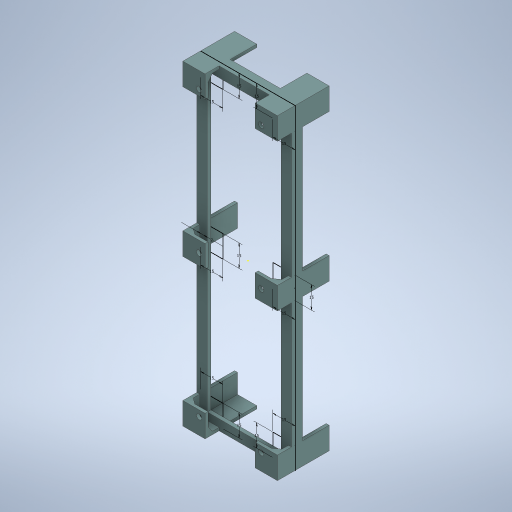
# Autodesk Inventor part: BaseMotor
Saved by Autodesk Inventor 2024 (Build 280153000, 153)
## iProperties
Created: 2024-02-15
Part Number: BaseMotor
Material: Generic
Document SubType Name: Modeling
Designer: fabiancastano
Density: 1 g/cm^3
Appearance: Default
Author: fabiancastano
Autodesk Inventor part; units mm, degrees
ref_plane "YZ Plane" through (0, 0, 0) normal (1, 0, 0) x (0, 1, 0)
ref_plane "XZ Plane" through (0, 0, 0) normal (0, 1, 0) x (-1, 0, 0)
ref_plane "XY Plane" through (0, 0, 0) normal (0, 0, 1) x (1, 0, 0)
sketch "Sketch1" plane through (0, 0, 0) normal (0, 0, 1) x (1, 0, 0)
  line L0 (-30, -105) -> (-30, 105) projected
  line L1 (-30, 105) -> (30, 105) projected
  line L2 (30, 105) -> (30, -105) projected
  line L3 (30, -105) -> (-30, -105) projected
  line L4 (-32, 107) -> (-32, -107)
  line L5 (-32, -107) -> (32, -107)
  line L6 (32, -107) -> (32, 107)
  line L7 (32, 107) -> (-32, 107)
  line L8 (-30, 105) -> (30, 105)
  line L9 (30, 105) -> (30, -105)
  line L10 (30, -105) -> (-30, -105)
  line L11 (-30, -105) -> (-30, 105)
  line L12 (-32, 107) -> (-17, 107)
  line L13 (-17, 107) -> (-17, 92)
  line L14 (-17, 92) -> (-32, 92)
  line L15 (-32, 92) -> (-32, 107)
  line L16 (32, 107) -> (17, 107)
  line L17 (17, 107) -> (17, 92)
  line L18 (17, 92) -> (32, 92)
  line L19 (32, 92) -> (32, 107)
  line L20 (32, -107) -> (17, -107)
  line L21 (17, -107) -> (17, -92)
  line L22 (17, -92) -> (32, -92)
  line L23 (32, -92) -> (32, -107)
  line L24 (-32, -107) -> (-17, -107)
  line L25 (-17, -107) -> (-17, -92)
  line L26 (-17, -92) -> (-32, -92)
  line L27 (-32, -92) -> (-32, -107)
  line L28 (17, 7.5) -> (32, 7.5)
  line L29 (32, 7.5) -> (32, -7.5)
  line L30 (32, -7.5) -> (17, -7.5)
  line L31 (17, -7.5) -> (17, 7.5)
  line L32 (-32, 7.5) -> (-17, 7.5)
  line L33 (-17, 7.5) -> (-17, -7.5)
  line L34 (-17, -7.5) -> (-32, -7.5)
  line L35 (-32, -7.5) -> (-32, 7.5)
  point P0 (0, 0)
  point P1 (-32, 0)
  point P2 (-32, 0)
  point P3 (32, 0)
  point P4 (32, 0)
  point P5 (-30, -7.5)
  point P6 (-30, 7.5)
  point P7 (30, -7.5)
  point P8 (30, 7.5)
  point P9 (-30, -92)
  point P10 (-17, -105)
  point P11 (30, -92)
  point P12 (17, -105)
  point P13 (30, 92)
  point P14 (17, 105)
  point P15 (-30, 92)
  point P16 (-17, 105)
  dimension "d0" = 2
  dimension "d1" = 15
  dimension "d2" = 15
  dimension "d3" = 15
  dimension "d4" = 15
  dimension "d5" = 15
  dimension "d6" = 15
  dimension "d7" = 15
  dimension "d8" = 15
  dimension "d9" = 15
  dimension "d10" = 15
  dimension "d11" = 15
  dimension "d12" = 15
  constraints: 64 end point, 14 parallel, 7 horizontal, 7 perpendicular, 4 coincident, 4 midpoint, 3 other
  measures "d0" distance between parallel lines of L0 L4
  measures "d1" distance of L13.end L14.end
  measures "d2" distance of L12.end L13.end
  measures "d3" distance of L18.end L17.end
  measures "d4" distance of L17.end L16.end
  measures "d5" distance of L21.end L22.end
  measures "d6" distance of L20.end L21.end
  measures "d7" distance of L26.end L25.end
  measures "d8" distance of L25.end L24.end
  measures "d9" distance of L29.end L30.end
  measures "d10" distance of L28.end L29.end
  measures "d11" distance of L33.end L34.end
  measures "d12" distance of L32.end L33.end
extrude "Extrusion1" add sketch "Sketch1" against normal blind 23 contours L3 L25 L5 L4 L26 L0 | L34 L4 L32 L0 | L3 L2 L22 L6 L5 L21 | L14 L4 L7 L13 L1 L0 | L2 L28 L6 L30 | L17 L7 L6 L18 L2 L1
sketch "Sketch2" plane through (0, 0, 0) normal (0, 0, 1) x (1, 0, 0)
  line L0 (17, 107) -> (17, 105) projected
  line L1 (17, 105) -> (17, 107) projected
  line L2 (17, 107) -> (17, 105) projected
  line L3 (17, 105) -> (17, 107) projected
  line L4 (30, 105) -> (17, 105) projected
  line L5 (17, 105) -> (30, 105) projected
  line L6 (30, 105) -> (17, 105) projected
  line L7 (30, 92) -> (30, 105) projected
  line L8 (30, 105) -> (30, 92) projected
  line L9 (30, 92) -> (30, 105) projected
  line L10 (17, 107) -> (32, 107) projected
  line L11 (32, 107) -> (17, 107) projected
  line L12 (17, 107) -> (32, 107) projected
  line L13 (32, 107) -> (32, 92) projected
  line L14 (32, 92) -> (32, 107) projected
  line L15 (32, 107) -> (32, 92) projected
  line L16 (32, 107) -> (32, 92) projected
  line L17 (32, 92) -> (30, 92) projected
  line L18 (30, 92) -> (30, 105) projected
  line L19 (30, 105) -> (17, 105) projected
  line L20 (17, 105) -> (17, 107) projected
  line L21 (17, 107) -> (32, 107) projected
  line L22 (17, 105) -> (30, 105) projected
  line L23 (32, 107) -> (17, 107) projected
  line L24 (32, 92) -> (32, 107) projected
  line L25 (32, 107) -> (17, 107) projected
  line L26 (17, 107) -> (17, 105) projected
  line L27 (17, 105) -> (30, 105) projected
  line L28 (30, 105) -> (30, 92) projected
  line L29 (30, 92) -> (32, 92) projected
  line L30 (32, 92) -> (32, 107) projected
  line L31 (-30, -7.5) -> (-30, 7.5) projected
  line L32 (-30, -7.5) -> (-30, 7.5) projected
  line L33 (-30, 7.5) -> (-30, -7.5) projected
  line L34 (-32, -7.5) -> (-30, -7.5) projected
  line L35 (-30, 7.5) -> (-32, 7.5) projected
  line L36 (-32, 7.5) -> (-32, -7.5) projected
  line L37 (-32, 7.5) -> (-32, -7.5) projected
  line L38 (-32, -7.5) -> (-32, 7.5) projected
  line L39 (-32, -7.5) -> (-30, -7.5) projected
  line L40 (-30, -7.5) -> (-32, -7.5) projected
  line L41 (-30, -7.5) -> (-30, 7.5) projected
  line L42 (-30, 7.5) -> (-32, 7.5) projected
  line L43 (-32, 7.5) -> (-32, -7.5) projected
  line L44 (-32, -7.5) -> (-30, -7.5) projected
  line L45 (-30, 7.5) -> (-32, 7.5) projected
  line L46 (-32, 7.5) -> (-30, 7.5) projected
  line L47 (-30, -7.5) -> (-32, -7.5) projected
  line L48 (-32, -7.5) -> (-32, 7.5) projected
  line L49 (-32, 7.5) -> (-30, 7.5) projected
  line L50 (-30, 7.5) -> (-30, -7.5) projected
  line L51 (-30, -7.5) -> (-32, -7.5) projected
  line L52 (-32, -7.5) -> (-32, 7.5) projected
  line L53 (-32, 7.5) -> (-30, 7.5) projected
  line L54 (-30, 7.5) -> (-30, -7.5) projected
  line L55 (17, -105) -> (17, -107) projected
  line L56 (17, -105) -> (17, -107) projected
  line L57 (17, -107) -> (17, -105) projected
  line L58 (17, -107) -> (17, -105) projected
  line L59 (30, -92) -> (30, -105) projected
  line L60 (30, -92) -> (30, -105) projected
  line L61 (30, -105) -> (30, -92) projected
  line L62 (30, -105) -> (17, -105) projected
  line L63 (30, -105) -> (17, -105) projected
  line L64 (17, -105) -> (30, -105) projected
  line L65 (32, -107) -> (32, -92) projected
  line L66 (32, -107) -> (32, -92) projected
  line L67 (32, -92) -> (32, -107) projected
  line L68 (17, -107) -> (32, -107) projected
  line L69 (30, -92) -> (30, -105) projected
  line L70 (30, -105) -> (17, -105) projected
  line L71 (17, -105) -> (17, -107) projected
  line L72 (17, -107) -> (32, -107) projected
  line L73 (32, -107) -> (32, -92) projected
  line L74 (32, -92) -> (30, -92) projected
  line L75 (17, -107) -> (32, -107) projected
  line L76 (32, -107) -> (17, -107) projected
  line L77 (30, -105) -> (30, -92) projected
  line L78 (17, -105) -> (30, -105) projected
  line L79 (32, -107) -> (17, -107) projected
  line L80 (30, -105) -> (30, -92) projected
  line L81 (30, -92) -> (32, -92) projected
  line L82 (32, -92) -> (32, -107) projected
  line L83 (32, -107) -> (17, -107) projected
  line L84 (17, -107) -> (17, -105) projected
  line L85 (17, -105) -> (30, -105) projected
  line L86 (32, -92) -> (32, -107) projected
  line L87 (30, 92) -> (32, 92) projected
  line L88 (32, 92) -> (30, 92) projected
  line L89 (30, 92) -> (32, 92) projected
  line L90 (32, 92) -> (30, 92) projected
  line L91 (30, 105) -> (30, 92) projected
  line L92 (-30, 105) -> (-30, 92) projected
  line L93 (-30, 92) -> (-30, 105) projected
  line L94 (-30, 92) -> (-32, 92) projected
  line L95 (-32, 92) -> (-30, 92) projected
  line L96 (-32, 92) -> (-32, 107) projected
  line L97 (-32, 107) -> (-32, 92) projected
  line L98 (-32, 107) -> (-17, 107) projected
  line L99 (-17, 107) -> (-32, 107) projected
  line L100 (-17, 107) -> (-17, 105) projected
  line L101 (-17, 105) -> (-17, 107) projected
  line L102 (-17, 105) -> (-17, 107) projected
  line L103 (-17, 107) -> (-17, 105) projected
  line L104 (-30, 105) -> (-17, 105) projected
  line L105 (-30, 92) -> (-30, 105) projected
  line L106 (-30, 105) -> (-17, 105) projected
  line L107 (-17, 105) -> (-17, 107) projected
  line L108 (-17, 107) -> (-32, 107) projected
  line L109 (-32, 107) -> (-32, 92) projected
  line L110 (-32, 92) -> (-30, 92) projected
  line L111 (-17, 105) -> (-30, 105) projected
  line L112 (-30, 105) -> (-17, 105) projected
  line L113 (-17, 105) -> (-30, 105) projected
  line L114 (-30, 92) -> (-30, 105) projected
  line L115 (-30, 105) -> (-30, 92) projected
  line L116 (-17, 107) -> (-32, 107) projected
  line L117 (-32, 107) -> (-17, 107) projected
  line L118 (-30, 105) -> (-30, 92) projected
  line L119 (-30, 92) -> (-32, 92) projected
  line L120 (-32, 92) -> (-32, 107) projected
  line L121 (-32, 107) -> (-17, 107) projected
  line L122 (-17, 107) -> (-17, 105) projected
  line L123 (-17, 105) -> (-30, 105) projected
  line L124 (-32, 107) -> (-32, 92) projected
  line L125 (-32, 92) -> (-32, 107) projected
  line L126 (-32, 92) -> (-30, 92) projected
  line L127 (-30, 92) -> (-32, 92) projected
  line L128 (30, -92) -> (32, -92) projected
  line L129 (32, -92) -> (30, -92) projected
  line L130 (32, -92) -> (30, -92) projected
  line L131 (30, -92) -> (32, -92) projected
  line L132 (-32, -107) -> (-32, -92) projected
  line L133 (-32, -92) -> (-32, -107) projected
  line L134 (-32, -92) -> (-30, -92) projected
  line L135 (-30, -92) -> (-32, -92) projected
  line L136 (-30, -92) -> (-30, -105) projected
  line L137 (-30, -105) -> (-30, -92) projected
  line L138 (-30, -105) -> (-17, -105) projected
  line L139 (-17, -105) -> (-30, -105) projected
  line L140 (-17, -105) -> (-17, -107) projected
  line L141 (-17, -107) -> (-17, -105) projected
  line L142 (-17, -107) -> (-17, -105) projected
  line L143 (-17, -105) -> (-17, -107) projected
  line L144 (-17, -107) -> (-32, -107) projected
  line L145 (-32, -107) -> (-32, -92) projected
  line L146 (-32, -92) -> (-30, -92) projected
  line L147 (-30, -92) -> (-30, -105) projected
  line L148 (-30, -105) -> (-17, -105) projected
  line L149 (-17, -105) -> (-17, -107) projected
  line L150 (-17, -107) -> (-32, -107) projected
  line L151 (-17, -105) -> (-30, -105) projected
  line L152 (-30, -105) -> (-17, -105) projected
  line L153 (-30, -105) -> (-30, -92) projected
  line L154 (-30, -92) -> (-30, -105) projected
  line L155 (-32, -107) -> (-17, -107) projected
  line L156 (-32, -107) -> (-17, -107) projected
  line L157 (-17, -107) -> (-32, -107) projected
  line L158 (-32, -92) -> (-32, -107) projected
  line L159 (-32, -107) -> (-17, -107) projected
  line L160 (-17, -107) -> (-17, -105) projected
  line L161 (-17, -105) -> (-30, -105) projected
  line L162 (-30, -105) -> (-30, -92) projected
  line L163 (-30, -92) -> (-32, -92) projected
  line L164 (-32, -92) -> (-32, -107) projected
  line L165 (-32, -107) -> (-32, -92) projected
  line L166 (-30, -92) -> (-32, -92) projected
  line L167 (-32, -92) -> (-30, -92) projected
  line L168 (32, 7.5) -> (32, -7.5) projected
  line L169 (32, -7.5) -> (32, 7.5) projected
  line L170 (30, -7.5) -> (30, 7.5) projected
  line L171 (32, -7.5) -> (30, -7.5) projected
  line L172 (30, 7.5) -> (32, 7.5) projected
  line L173 (32, 7.5) -> (32, -7.5) projected
  line L174 (32, -7.5) -> (30, -7.5) projected
  line L175 (30, -7.5) -> (30, 7.5) projected
  line L176 (30, 7.5) -> (32, 7.5) projected
  line L177 (30, 7.5) -> (30, -7.5) projected
  line L178 (30, 7.5) -> (30, -7.5) projected
  line L179 (30, -7.5) -> (30, 7.5) projected
  line L180 (32, 7.5) -> (30, 7.5) projected
  line L181 (32, 7.5) -> (30, 7.5) projected
  line L182 (30, 7.5) -> (32, 7.5) projected
  line L183 (32, -7.5) -> (32, 7.5) projected
  line L184 (32, 7.5) -> (30, 7.5) projected
  line L185 (30, 7.5) -> (30, -7.5) projected
  line L186 (30, -7.5) -> (32, -7.5) projected
  line L187 (32, -7.5) -> (32, 7.5) projected
  line L188 (32, 7.5) -> (32, -7.5) projected
  line L189 (30, -7.5) -> (32, -7.5) projected
  line L190 (30, -7.5) -> (32, -7.5) projected
  line L191 (32, -7.5) -> (30, -7.5) projected
  line L192 (-32, -7.5) -> (-32, 7.5) projected
  line L193 (-32, 7.5) -> (-17, 7.5) projected
  line L194 (-17, 7.5) -> (-17, -7.5) projected
  line L195 (17, -7.5) -> (17, 7.5) projected
  line L196 (32, -7.5) -> (17, -7.5) projected
  line L197 (17, 7.5) -> (32, 7.5) projected
  line L198 (32, 7.5) -> (32, -7.5) projected
  line L199 (30, 105) -> (30, -105) projected
  line L200 (30, 105) -> (30, -105) projected
  line L201 (32, -107) -> (32, 107) projected
  line L202 (-30, -105) -> (-30, 105) projected
  line L203 (-30, -105) -> (-30, 105) projected
  line L204 (-32, 107) -> (-32, -107) projected
  line L205 (-30, 105) -> (30, 105) projected
  line L206 (32, 107) -> (-32, 107) projected
  line L207 (-30, 105) -> (30, 105) projected
  line L208 (-17, 92) -> (-32, 92) projected
  line L209 (-32, 107) -> (-17, 107) projected
  line L210 (-32, 92) -> (-32, 107) projected
  line L211 (-17, 107) -> (-17, 92) projected
  line L212 (17, 92) -> (32, 92) projected
  line L213 (17, 107) -> (17, 92) projected
  line L214 (32, 107) -> (17, 107) projected
  line L215 (32, 92) -> (32, 107) projected
  line L216 (30, -105) -> (-30, -105) projected
  line L217 (-32, -107) -> (32, -107) projected
  line L218 (30, -105) -> (-30, -105) projected
  line L219 (-17, -92) -> (-32, -92) projected
  line L220 (-32, -92) -> (-32, -107) projected
  line L221 (-32, -107) -> (-17, -107) projected
  line L222 (-17, -107) -> (-17, -92) projected
  line L223 (17, -92) -> (32, -92) projected
  line L224 (17, -107) -> (17, -92) projected
  line L225 (32, -92) -> (32, -107) projected
  line L226 (32, -107) -> (17, -107) projected
  line L227 (-17, -7.5) -> (-32, -7.5) projected
  point P0 (0, 0)
  point P1 (0, 0)
  point P2 (32, 0)
  point P3 (32, 0)
  point P4 (-32, 0)
  point P5 (-32, 0)
  constraints: 51 other
extrude "Extrusion2" add sketch "Sketch2" against normal blind 5 contours L0 L205 L100 L206 | L201 L172 L199 L17 | L94 L202 L35 L204 | L201 L74 L199 L171 | L34 L202 L134 L204 | L217 L140 L216 L55
sketch "Sketch5" plane through (0, 0, 0) normal (0, 0, 1) x (1, 0, 0)
  line L0 (17, 107) -> (32, 107) projected
  line L1 (-32, -107) -> (32, -107) projected
  line L2 (32, 107) -> (-32, 107)
  line L3 (-32, 107) -> (-32, -107)
  line L4 (-32, -107) -> (32, -107)
  line L5 (32, -107) -> (32, 107)
  line L6 (25, 100) -> (-25, 100)
  line L7 (-25, 100) -> (-25, -100)
  line L8 (-25, -100) -> (25, -100)
  line L9 (25, -100) -> (25, 100)
  point P0 (0, 0)
  point P1 (32, -107)
  dimension "d17" = 7
  constraints: 16 end point, 4 parallel, 2 perpendicular, 1 horizontal, 3 other
  measures "d17" distance between parallel lines of L5 L9
extrude "Extrusion3" add sketch "Sketch5" along normal blind 2.5
sketch "Sketch6" plane through (0, 0, 0) normal (0, 0, -1) x (-1, 0, 0)
  line L0 (32, 7.5) -> (32, 92) projected
  line L1 (32, 92) -> (32, 107) projected
  line L2 (-17, 107) -> (-32, 107) projected
  line L3 (30, 7.5) -> (30, -7.5) projected
  line L4 (32, -7.5) -> (32, 7.5) projected
  line L5 (30, 7.5) -> (30, -7.5) projected
  line L6 (30, -7.5) -> (32, -7.5) projected
  line L7 (32, -7.5) -> (32, 7.5) projected
  line L8 (32, 7.5) -> (30, 7.5) projected
  line L9 (-30, -7.5) -> (-30, 7.5) projected
  line L10 (25, -100) -> (25, 100) projected
  line L11 (-32, 107) -> (-32, 92) projected
  line L12 (-32, 92) -> (-32, 7.5) projected
  line L13 (17, -107) -> (32, -107) projected
  line L14 (-32, -92) -> (-32, -107) projected
  line L15 (30, -7.5) -> (30, -92) projected
  line L16 (-32, -7.5) -> (-32, -92) projected
  line L17 (32, -92) -> (32, -7.5) projected
  line L18 (-32, 7.5) -> (-32, -7.5) projected
  line L19 (-32, 7.5) -> (-32, -7.5) projected
  line L20 (-32, -7.5) -> (-30, -7.5) projected
  line L21 (-30, -7.5) -> (-30, 7.5) projected
  line L22 (-30, 7.5) -> (-32, 7.5) projected
  line L23 (-25, 100) -> (-25, -100) projected
  line L24 (-25, 100) -> (-25, -100) projected
  line L25 (-25, 100) -> (-25, -100) projected
  line L26 (-25, 100) -> (-25, -100) projected
  line L27 (-30, 105) -> (-30, -105) projected
  line L28 (-30, 92) -> (-30, 105) projected
  line L29 (-30, 7.5) -> (-30, 92) projected
  line L30 (-30, -7.5) -> (-30, 7.5) projected
  line L31 (-30, -92) -> (-30, -7.5) projected
  line L32 (-30, -105) -> (-30, -92) projected
  line L33 (-30, 105) -> (-30, -105) projected
  line L34 (-25, 100) -> (-25, -100) projected
  line L35 (25, 100) -> (-25, 100) projected
  line L36 (25, -100) -> (25, 100) projected
  line L37 (-25, -100) -> (25, -100) projected
  line L38 (30, 105) -> (-30, 105) projected
  line L39 (-30, 105) -> (-30, -105) projected
  line L40 (-30, -105) -> (30, -105) projected
  line L41 (30, -105) -> (30, 105) projected
  line L42 (-32, -92) -> (-32, -107) projected
  line L43 (-32, -7.5) -> (-32, -92) projected
  line L44 (-32, 7.5) -> (-32, -7.5) projected
  line L45 (-32, 92) -> (-32, 7.5) projected
  line L46 (-32, 107) -> (-32, 92) projected
  line L47 (-32, -107) -> (-32, 107) projected
  line L48 (-32, -107) -> (-32, 107) projected
  line L49 (32, -107) -> (-32, -107) projected
  line L50 (-32, -107) -> (-32, 107) projected
  line L51 (-32, 107) -> (32, 107) projected
  line L52 (32, 107) -> (32, -107) projected
  line L53 (-25, 100) -> (-25, -100) projected
  line L54 (-25, -100) -> (25, -100) projected
  line L55 (25, -100) -> (25, 100) projected
  line L56 (25, 100) -> (-25, 100) projected
  line L57 (17, 107) -> (-17, 107) projected
  line L58 (30, -105) -> (30, 105) projected
  line L59 (30, -105) -> (30, 105) projected
  line L60 (30, -92) -> (30, -105) projected
  line L61 (30, -7.5) -> (30, -92) projected
  line L62 (30, 7.5) -> (30, -7.5) projected
  line L63 (30, 92) -> (30, 7.5) projected
  line L64 (30, 105) -> (30, 92) projected
  line L65 (32, 107) -> (32, -107) projected
  line L66 (32, 92) -> (32, 107) projected
  line L67 (32, 7.5) -> (32, 92) projected
  line L68 (32, -7.5) -> (32, 7.5) projected
  line L69 (32, -92) -> (32, -7.5) projected
  line L70 (32, -107) -> (32, -92) projected
  line L71 (32, 107) -> (32, -107) projected
  line L72 (32, 107) -> (17, 107) projected
  line L73 (25, -100) -> (25, 100) projected
  line L74 (25, -100) -> (25, 100) projected
  line L75 (25, -100) -> (25, 100) projected
  line L76 (-30, -92) -> (-30, -7.5) projected
  line L77 (-30, -105) -> (-30, -92) projected
  line L78 (-32, -107) -> (-17, -107) projected
  line L79 (-17, -107) -> (-17, -105) projected
  line L80 (-30, -92) -> (-32, -92) projected
  line L81 (-25, -100) -> (25, -100) projected
  line L82 (-25, -100) -> (25, -100) projected
  line L83 (-25, -100) -> (25, -100) projected
  line L84 (-25, -100) -> (25, -100) projected
  line L85 (17, -105) -> (-17, -105) projected
  line L86 (-17, -107) -> (17, -107) projected
  line L87 (-17, -105) -> (-30, -105) projected
  line L88 (-30, -105) -> (30, -105) projected
  line L89 (-17, -105) -> (-30, -105) projected
  line L90 (17, -105) -> (-17, -105) projected
  line L91 (30, -105) -> (17, -105) projected
  line L92 (-30, -105) -> (30, -105) projected
  line L93 (32, -107) -> (-32, -107) projected
  line L94 (17, -107) -> (32, -107) projected
  line L95 (-17, -107) -> (17, -107) projected
  line L96 (-32, -107) -> (-17, -107) projected
  line L97 (32, -107) -> (-32, -107) projected
  line L98 (-32, -7.5) -> (-30, -7.5) projected
  line L99 (30, -7.5) -> (32, -7.5) projected
  line L100 (30, -7.5) -> (32, -7.5) projected
  line L101 (-32, -7.5) -> (-30, -7.5) projected
  line L102 (-32, -7.5) -> (-30, -7.5) projected
  line L103 (-32, -7.5) -> (-30, -7.5) projected
  line L104 (32, -92) -> (30, -92) projected
  line L105 (32, -92) -> (32, -7.5) projected
  line L106 (30, -7.5) -> (32, -7.5) projected
  line L107 (30, -7.5) -> (30, -92) projected
  line L108 (-32, -7.5) -> (-30, -7.5) projected
  line L109 (-32, -7.5) -> (-32, -92) projected
  line L110 (-30, -92) -> (-32, -92) projected
  line L111 (-30, -92) -> (-30, -7.5) projected
  line L112 (32, -92) -> (30, -92) projected
  line L113 (32, -92) -> (30, -92) projected
  line L114 (-30, -92) -> (-32, -92) projected
  line L115 (-30, -92) -> (-32, -92) projected
  line L116 (-30, -92) -> (-32, -92) projected
  line L117 (32, -107) -> (32, -92) projected
  line L118 (32, -92) -> (30, -92) projected
  line L119 (30, -92) -> (30, -105) projected
  line L120 (30, -105) -> (17, -105) projected
  line L121 (17, -105) -> (17, -107) projected
  line L122 (17, -107) -> (32, -107) projected
  line L123 (-30, -105) -> (-30, -92) projected
  line L124 (-30, -92) -> (-32, -92) projected
  line L125 (-32, -92) -> (-32, -107) projected
  line L126 (-32, -107) -> (-17, -107) projected
  line L127 (-17, -107) -> (-17, -105) projected
  line L128 (-17, -105) -> (-30, -105) projected
  line L129 (-17, -107) -> (-17, -105) projected
  line L130 (-17, -107) -> (-17, -105) projected
  line L131 (-17, -107) -> (-17, -105) projected
  line L132 (-17, -107) -> (17, -107) projected
  line L133 (17, -105) -> (17, -107) projected
  line L134 (17, -105) -> (-17, -105) projected
  line L135 (17, -105) -> (17, -107) projected
  line L136 (17, -105) -> (17, -107) projected
  line L137 (30, -105) -> (17, -105) projected
  line L138 (30, -92) -> (30, -105) projected
  line L139 (32, -107) -> (32, -92) projected
  line L140 (30, -7.5) -> (32, -7.5) projected
  line L141 (30, -7.5) -> (32, -7.5) projected
  line L142 (32, -92) -> (30, -92) projected
  line L143 (32, -92) -> (30, -92) projected
  line L144 (-17, -107) -> (-17, -105) projected
  line L145 (17, -105) -> (17, -107) projected
  line L146 (17, -105) -> (17, -107) projected
  line L147 (17, 107) -> (17, 105) projected
  line L148 (17, 107) -> (17, 105) projected
  line L149 (17, 107) -> (17, 105) projected
  line L150 (32, 7.5) -> (30, 7.5) projected
  line L151 (-30, 7.5) -> (-32, 7.5) projected
  line L152 (-30, 7.5) -> (-32, 7.5) projected
  line L153 (30, 92) -> (30, 7.5) projected
  line L154 (30, 105) -> (30, 92) projected
  line L155 (17, 105) -> (30, 105) projected
  line L156 (-30, 7.5) -> (-32, 7.5) projected
  line L157 (32, 7.5) -> (30, 7.5) projected
  line L158 (-30, 7.5) -> (-32, 7.5) projected
  line L159 (32, 7.5) -> (30, 7.5) projected
  line L160 (32, 7.5) -> (30, 7.5) projected
  line L161 (32, 7.5) -> (30, 7.5) projected
  line L162 (32, 7.5) -> (32, 92) projected
  line L163 (30, 92) -> (32, 92) projected
  line L164 (30, 92) -> (30, 7.5) projected
  line L165 (-32, 92) -> (-30, 92) projected
  line L166 (-32, 92) -> (-32, 7.5) projected
  line L167 (-30, 7.5) -> (-32, 7.5) projected
  line L168 (-30, 7.5) -> (-30, 92) projected
  line L169 (25, 100) -> (-25, 100) projected
  line L170 (30, 105) -> (-30, 105) projected
  line L171 (30, 105) -> (-30, 105) projected
  line L172 (17, 105) -> (30, 105) projected
  line L173 (-17, 105) -> (17, 105) projected
  line L174 (-30, 105) -> (-17, 105) projected
  line L175 (-17, 107) -> (-32, 107) projected
  line L176 (17, 107) -> (-17, 107) projected
  line L177 (32, 107) -> (17, 107) projected
  line L178 (-32, 107) -> (32, 107) projected
  line L179 (-32, 107) -> (32, 107) projected
  line L180 (25, 100) -> (-25, 100) projected
  line L181 (17, 107) -> (17, 105) projected
  line L182 (30, 92) -> (32, 92) projected
  line L183 (30, 105) -> (30, 92) projected
  line L184 (30, 92) -> (32, 92) projected
  line L185 (32, 92) -> (32, 107) projected
  line L186 (32, 107) -> (17, 107) projected
  line L187 (17, 107) -> (17, 105) projected
  line L188 (17, 105) -> (30, 105) projected
  line L189 (30, 92) -> (32, 92) projected
  line L190 (30, 92) -> (32, 92) projected
  line L191 (30, 92) -> (32, 92) projected
  line L192 (25, 100) -> (-25, 100) projected
  line L193 (25, 100) -> (-25, 100) projected
  line L194 (17, 107) -> (17, 105) projected
  line L195 (17, 107) -> (-17, 107) projected
  line L196 (-17, 105) -> (-17, 107) projected
  line L197 (-17, 105) -> (17, 105) projected
  line L198 (-17, 105) -> (17, 105) projected
  line L199 (-30, 105) -> (-17, 105) projected
  line L200 (-30, 92) -> (-30, 105) projected
  line L201 (-17, 105) -> (-17, 107) projected
  line L202 (-32, 92) -> (-30, 92) projected
  line L203 (-32, 92) -> (-30, 92) projected
  line L204 (-32, 92) -> (-30, 92) projected
  line L205 (-32, 92) -> (-30, 92) projected
  line L206 (-32, 107) -> (-32, 92) projected
  line L207 (-32, 92) -> (-30, 92) projected
  line L208 (-30, 92) -> (-30, 105) projected
  line L209 (-30, 105) -> (-17, 105) projected
  line L210 (-17, 105) -> (-17, 107) projected
  line L211 (-17, 107) -> (-32, 107) projected
  line L212 (-17, 105) -> (-17, 107) projected
  line L213 (-17, 105) -> (-17, 107) projected
  line L214 (-17, 105) -> (-17, 107) projected
  line L215 (-30, 7.5) -> (-30, 92) projected
  line L216 (32, -7.5) -> (32, 7.5) projected
  line L217 (32, 7.5) -> (17, 7.5) projected
  line L218 (17, 7.5) -> (17, -7.5) projected
  line L219 (-17, -7.5) -> (-17, 7.5) projected
  line L220 (-32, -7.5) -> (-17, -7.5) projected
  line L221 (-17, 7.5) -> (-32, 7.5) projected
  line L222 (-32, 7.5) -> (-32, -7.5) projected
  line L223 (-30, 105) -> (-30, -105) projected
  line L224 (-30, 105) -> (-30, -105) projected
  line L225 (-32, -107) -> (-32, 107) projected
  line L226 (30, -105) -> (30, 105) projected
  line L227 (30, -105) -> (30, 105) projected
  line L228 (32, 107) -> (32, -107) projected
  line L229 (30, 105) -> (-30, 105) projected
  line L230 (-32, 107) -> (32, 107) projected
  line L231 (30, 105) -> (-30, 105) projected
  line L232 (17, 92) -> (32, 92) projected
  line L233 (32, 107) -> (17, 107) projected
  line L234 (32, 92) -> (32, 107) projected
  line L235 (17, 107) -> (17, 92) projected
  line L236 (-17, 92) -> (-32, 92) projected
  line L237 (-17, 107) -> (-17, 92) projected
  line L238 (-32, 107) -> (-17, 107) projected
  line L239 (-32, 92) -> (-32, 107) projected
  line L240 (-30, -105) -> (30, -105) projected
  line L241 (32, -107) -> (-32, -107) projected
  line L242 (-30, -105) -> (30, -105) projected
  line L243 (17, -92) -> (32, -92) projected
  line L244 (32, -92) -> (32, -107) projected
  line L245 (32, -107) -> (17, -107) projected
  line L246 (17, -107) -> (17, -92) projected
  line L247 (-17, -92) -> (-32, -92) projected
  line L248 (-17, -107) -> (-17, -92) projected
  line L249 (-32, -92) -> (-32, -107) projected
  line L250 (-32, -107) -> (-17, -107) projected
  line L251 (17, -7.5) -> (32, -7.5) projected
  point P0 (0, 0)
  point P1 (0, 0)
  point P2 (-32, 0)
  point P3 (-32, 0)
  point P4 (32, 0)
  point P5 (32, 0)
  constraints: 72 other
extrude "Extrusion4" add sketch "Sketch6" against normal blind 10 contours L4 L6 L3 L8 | L163 L41 L38 L147 L51 L1 | L52 L13 L121 L40 L41 L104 | L196 L38 L27 L165 L11 L2 | L49 L14 L80 L27 L40 L79 | L22 L9 L20 L18
sketch "Sketch7" plane through (0, 0, 10) normal (0, 0, 1) x (1, 0, 0)
  line L0 (-30, -7.5) -> (-32, -7.5) projected
  line L1 (-32, 7.5) -> (-32, -7.5) projected
  line L2 (-30, 7.5) -> (-30, -7.5) projected
  line L3 (-30, -7.5) -> (-30, 7.5) projected
  line L4 (-30, 7.5) -> (-30, -7.5) projected
  line L5 (-30, -7.5) -> (-30, 7.5) projected
  line L6 (30, -7.5) -> (30, 7.5) projected
  line L7 (32, 7.5) -> (32, -7.5) projected
  line L8 (32, -7.5) -> (30, -7.5) projected
  line L9 (30, -7.5) -> (30, 7.5) projected
  line L10 (30, 7.5) -> (32, 7.5) projected
  line L11 (30, -7.5) -> (30, 7.5) projected
  line L12 (30, -7.5) -> (30, 7.5) projected
  line L13 (30, 7.5) -> (30, -7.5) projected
  line L14 (32, -7.5) -> (30, -7.5) projected
  line L15 (32, -7.5) -> (30, -7.5) projected
  line L16 (30, -7.5) -> (32, -7.5) projected
  line L17 (-30, -7.5) -> (-30, -92) projected
  line L18 (30, -92) -> (30, -7.5) projected
  line L19 (-30, -7.5) -> (-32, -7.5) projected
  line L20 (-30, -7.5) -> (-32, -7.5) projected
  line L21 (-32, -92) -> (-30, -92) projected
  line L22 (-32, -92) -> (-30, -92) projected
  line L23 (17, -107) -> (17, -105) projected
  line L24 (-17, -105) -> (-17, -107) projected
  line L25 (-17, -105) -> (-17, -107) projected
  line L26 (17, -107) -> (17, -105) projected
  line L27 (17, -105) -> (17, -107) projected
  line L28 (-17, -105) -> (-17, -107) projected
  line L29 (-17, -107) -> (-17, -105) projected
  line L30 (25, -100) -> (-25, -100) projected
  line L31 (25, -100) -> (-25, -100) projected
  line L32 (-32, -92) -> (-30, -92) projected
  line L33 (-30, -92) -> (-32, -92) projected
  line L34 (-30, -92) -> (-30, -105) projected
  line L35 (-30, -105) -> (-30, -92) projected
  line L36 (-32, -92) -> (-32, -107) projected
  line L37 (-30, -105) -> (-17, -105) projected
  line L38 (17, -107) -> (17, -105) projected
  line L39 (30, -105) -> (30, -92) projected
  line L40 (-32, -7.5) -> (-30, -7.5) projected
  line L41 (-30, -7.5) -> (-32, -7.5) projected
  line L42 (-32, -7.5) -> (-30, -7.5) projected
  line L43 (32, -7.5) -> (32, -92) projected
  line L44 (32, -92) -> (32, -7.5) projected
  line L45 (-32, -92) -> (-32, -7.5) projected
  line L46 (-32, -7.5) -> (-32, -92) projected
  line L47 (32, -92) -> (32, -107) projected
  line L48 (17, -107) -> (-17, -107) projected
  line L49 (-32, -107) -> (-32, -92) projected
  line L50 (-17, -107) -> (-32, -107) projected
  line L51 (-17, -107) -> (17, -107) projected
  line L52 (30, -105) -> (30, -92) projected
  line L53 (30, -92) -> (30, -105) projected
  line L54 (17, -105) -> (30, -105) projected
  line L55 (30, -105) -> (17, -105) projected
  line L56 (-30, -105) -> (-17, -105) projected
  line L57 (-17, -105) -> (-30, -105) projected
  line L58 (-30, -92) -> (-30, -105) projected
  line L59 (-30, -105) -> (-30, -92) projected
  line L60 (-32, -107) -> (-17, -107) projected
  line L61 (-17, -107) -> (-17, -105) projected
  line L62 (-17, -105) -> (-30, -105) projected
  line L63 (-30, -105) -> (-30, -92) projected
  line L64 (-30, -92) -> (-32, -92) projected
  line L65 (-32, -92) -> (-32, -107) projected
  line L66 (32, -107) -> (32, -92) projected
  line L67 (32, -92) -> (30, -92) projected
  line L68 (30, -92) -> (30, -105) projected
  line L69 (30, -105) -> (17, -105) projected
  line L70 (17, -105) -> (17, -107) projected
  line L71 (17, -107) -> (32, -107) projected
  line L72 (32, -7.5) -> (30, -7.5) projected
  line L73 (-30, -7.5) -> (-32, -7.5) projected
  line L74 (-30, -7.5) -> (-32, -7.5) projected
  line L75 (32, -7.5) -> (30, -7.5) projected
  line L76 (32, -7.5) -> (30, -7.5) projected
  line L77 (32, -7.5) -> (30, -7.5) projected
  line L78 (-32, -92) -> (-30, -92) projected
  line L79 (-32, -92) -> (-32, -7.5) projected
  line L80 (-30, -7.5) -> (-32, -7.5) projected
  line L81 (-30, -7.5) -> (-30, -92) projected
  line L82 (32, -7.5) -> (30, -7.5) projected
  line L83 (32, -7.5) -> (32, -92) projected
  line L84 (30, -92) -> (32, -92) projected
  line L85 (30, -92) -> (30, -7.5) projected
  line L86 (-32, -92) -> (-30, -92) projected
  line L87 (-32, -92) -> (-30, -92) projected
  line L88 (30, -92) -> (32, -92) projected
  line L89 (30, -92) -> (32, -92) projected
  line L90 (30, -92) -> (32, -92) projected
  line L91 (-32, -107) -> (-32, -92) projected
  line L92 (-32, -92) -> (-30, -92) projected
  line L93 (-30, -92) -> (-30, -105) projected
  line L94 (-30, -105) -> (-17, -105) projected
  line L95 (-17, -105) -> (-17, -107) projected
  line L96 (-17, -107) -> (-32, -107) projected
  line L97 (30, -105) -> (30, -92) projected
  line L98 (30, -92) -> (32, -92) projected
  line L99 (32, -92) -> (32, -107) projected
  line L100 (32, -107) -> (17, -107) projected
  line L101 (17, -107) -> (17, -105) projected
  line L102 (17, -105) -> (30, -105) projected
  line L103 (17, -107) -> (17, -105) projected
  line L104 (17, -107) -> (17, -105) projected
  line L105 (17, -107) -> (17, -105) projected
  line L106 (17, -107) -> (-17, -107) projected
  line L107 (-17, -105) -> (-17, -107) projected
  line L108 (-17, -105) -> (17, -105) projected
  line L109 (-17, -105) -> (-17, -107) projected
  line L110 (-17, -105) -> (-17, -107) projected
  line L111 (-30, 7.5) -> (-30, -7.5) projected
  line L112 (-32, -7.5) -> (-32, 7.5) projected
  line L113 (-30, -7.5) -> (-30, 7.5) projected
  line L114 (-30, 7.5) -> (-32, 7.5) projected
  line L115 (-32, 7.5) -> (-32, -7.5) projected
  line L116 (-32, -7.5) -> (-30, -7.5) projected
  line L117 (32, 7.5) -> (32, -7.5) projected
  line L118 (-30, 92) -> (-30, 7.5) projected
  line L119 (-25, 100) -> (25, 100) projected
  line L120 (-30, -92) -> (-30, -105) projected
  line L121 (-30, -105) -> (-17, -105) projected
  line L122 (25, -100) -> (-25, -100) projected
  line L123 (-17, -105) -> (17, -105) projected
  line L124 (25, -100) -> (-25, -100) projected
  line L125 (17, -105) -> (30, -105) projected
  line L126 (30, -105) -> (-30, -105) projected
  line L127 (-25, -100) -> (-25, 100) projected
  line L128 (-25, -100) -> (-25, 100) projected
  line L129 (-25, -100) -> (-25, 100) projected
  line L130 (-25, -100) -> (-25, 100) projected
  line L131 (25, 100) -> (25, -100) projected
  line L132 (25, 100) -> (25, -100) projected
  line L133 (25, 100) -> (25, -100) projected
  line L134 (25, 100) -> (25, -100) projected
  line L135 (-30, -105) -> (-30, 105) projected
  line L136 (-30, -105) -> (-30, 105) projected
  line L137 (-30, -92) -> (-30, -105) projected
  line L138 (-30, -7.5) -> (-30, -92) projected
  line L139 (-30, 7.5) -> (-30, -7.5) projected
  line L140 (-30, 92) -> (-30, 7.5) projected
  line L141 (-30, 105) -> (-30, 92) projected
  line L142 (-32, 92) -> (-32, 7.5) projected
  line L143 (-32, 107) -> (-32, 92) projected
  line L144 (-32, 92) -> (-32, 107) projected
  line L145 (-32, 7.5) -> (-32, 92) projected
  line L146 (-32, -7.5) -> (-32, 7.5) projected
  line L147 (-32, -92) -> (-32, -7.5) projected
  line L148 (-32, -107) -> (-32, -92) projected
  line L149 (-32, -92) -> (-32, -107) projected
  line L150 (-32, -7.5) -> (-32, -92) projected
  line L151 (-32, 7.5) -> (-32, -7.5) projected
  line L152 (25, 100) -> (25, -100) projected
  line L153 (-25, 100) -> (25, 100) projected
  line L154 (-25, -100) -> (-25, 100) projected
  line L155 (25, -100) -> (-25, -100) projected
  line L156 (-30, 105) -> (30, 105) projected
  line L157 (30, 105) -> (30, -105) projected
  line L158 (30, -105) -> (-30, -105) projected
  line L159 (-30, -105) -> (-30, 105) projected
  line L160 (-30, 92) -> (-32, 92) projected
  line L161 (-32, 92) -> (-32, 7.5) projected
  line L162 (-32, 7.5) -> (-30, 7.5) projected
  line L163 (-30, 7.5) -> (-30, -7.5) projected
  line L164 (-30, -7.5) -> (-32, -7.5) projected
  line L165 (-32, -7.5) -> (-32, -92) projected
  line L166 (-32, -92) -> (-30, -92) projected
  line L167 (-30, -92) -> (-30, -105) projected
  line L168 (-30, -105) -> (-17, -105) projected
  line L169 (-17, -105) -> (-17, -107) projected
  line L170 (-17, -107) -> (17, -107) projected
  line L171 (17, -107) -> (17, -105) projected
  line L172 (17, -105) -> (30, -105) projected
  line L173 (30, -105) -> (30, -92) projected
  line L174 (30, -92) -> (32, -92) projected
  line L175 (32, -92) -> (32, -7.5) projected
  line L176 (32, -7.5) -> (30, -7.5) projected
  line L177 (30, -7.5) -> (30, 7.5) projected
  line L178 (30, 7.5) -> (32, 7.5) projected
  line L179 (32, 7.5) -> (32, 92) projected
  line L180 (32, 92) -> (30, 92) projected
  line L181 (30, 92) -> (30, 105) projected
  line L182 (30, 105) -> (17, 105) projected
  line L183 (17, 105) -> (17, 107) projected
  line L184 (17, 107) -> (-17, 107) projected
  line L185 (-17, 107) -> (-17, 105) projected
  line L186 (-17, 105) -> (-30, 105) projected
  line L187 (-30, 105) -> (-30, 92) projected
  line L188 (25, 100) -> (25, -100) projected
  line L189 (25, -100) -> (-25, -100) projected
  line L190 (-25, -100) -> (-25, 100) projected
  line L191 (-25, 100) -> (25, 100) projected
  line L192 (30, 105) -> (30, -105) projected
  line L193 (30, 105) -> (30, -105) projected
  line L194 (30, 92) -> (30, 105) projected
  line L195 (30, 7.5) -> (30, 92) projected
  line L196 (30, -7.5) -> (30, 7.5) projected
  line L197 (30, -92) -> (30, -7.5) projected
  line L198 (30, -105) -> (30, -92) projected
  line L199 (32, -92) -> (32, -7.5) projected
  line L200 (32, -107) -> (32, -92) projected
  line L201 (32, -92) -> (32, -107) projected
  line L202 (32, -7.5) -> (32, -92) projected
  line L203 (32, 7.5) -> (32, -7.5) projected
  line L204 (32, 92) -> (32, 7.5) projected
  line L205 (32, 107) -> (32, 92) projected
  line L206 (32, 92) -> (32, 107) projected
  line L207 (32, 7.5) -> (32, 92) projected
  line L208 (32, -7.5) -> (32, 7.5) projected
  line L209 (-32, -92) -> (-30, -92) projected
  line L210 (-30, -92) -> (-32, -92) projected
  line L211 (-17, -107) -> (-17, -105) projected
  line L212 (-17, -105) -> (-17, -107) projected
  line L213 (-32, -107) -> (-17, -107) projected
  line L214 (17, -105) -> (17, -107) projected
  line L215 (30, -105) -> (17, -105) projected
  line L216 (30, -92) -> (30, -105) projected
  line L217 (32, -107) -> (32, -92) projected
  line L218 (30, -105) -> (-30, -105) projected
  line L219 (17, -105) -> (30, -105) projected
  line L220 (-17, -105) -> (17, -105) projected
  line L221 (-30, -105) -> (-17, -105) projected
  line L222 (17, -107) -> (32, -107) projected
  line L223 (-17, -107) -> (17, -107) projected
  line L224 (-32, -107) -> (-17, -107) projected
  line L225 (-17, -107) -> (-32, -107) projected
  line L226 (17, -107) -> (-17, -107) projected
  line L227 (32, -107) -> (17, -107) projected
  line L228 (17, -107) -> (32, -107) projected
  line L229 (-17, -105) -> (-30, -105) projected
  line L230 (30, -105) -> (30, -92) projected
  line L231 (32, -107) -> (17, -107) projected
  line L232 (17, -107) -> (17, -105) projected
  line L233 (30, -92) -> (32, -92) projected
  line L234 (17, -105) -> (30, -105) projected
  line L235 (32, -92) -> (30, -92) projected
  line L236 (30, -92) -> (32, -92) projected
  line L237 (30, -92) -> (32, -92) projected
  line L238 (32, -92) -> (30, -92) projected
  line L239 (30, -7.5) -> (32, -7.5) projected
  line L240 (30, 7.5) -> (30, -7.5) projected
  line L241 (32, -7.5) -> (32, 7.5) projected
  line L242 (32, -7.5) -> (32, 7.5) projected
  line L243 (32, 7.5) -> (30, 7.5) projected
  line L244 (30, 7.5) -> (30, -7.5) projected
  line L245 (30, -7.5) -> (32, -7.5) projected
  line L246 (-30, 7.5) -> (-30, -7.5) projected
  line L247 (-30, -7.5) -> (-32, -7.5) projected
  line L248 (-32, -7.5) -> (-32, 7.5) projected
  line L249 (-32, 7.5) -> (-30, 7.5) projected
  line L250 (30, 7.5) -> (32, 7.5) projected
  line L251 (32, 92) -> (32, 7.5) projected
  line L252 (32, 92) -> (30, 92) projected
  line L253 (30, 105) -> (17, 105) projected
  line L254 (30, 92) -> (30, 105) projected
  line L255 (-30, 105) -> (-30, 92) projected
  line L256 (-17, 105) -> (-30, 105) projected
  line L257 (-17, 107) -> (-17, 105) projected
  line L258 (30, 7.5) -> (30, 92) projected
  line L259 (30, 92) -> (30, 105) projected
  line L260 (-30, 105) -> (-30, 92) projected
  line L261 (30, 105) -> (17, 105) projected
  line L262 (32, 7.5) -> (32, 92) projected
  line L263 (-25, 100) -> (25, 100) projected
  line L264 (-30, 105) -> (30, 105) projected
  line L265 (32, 107) -> (32, 92) projected
  line L266 (17, 107) -> (32, 107) projected
  line L267 (17, 105) -> (-17, 105) projected
  line L268 (17, 107) -> (-17, 107) projected
  line L269 (-17, 107) -> (17, 107) projected
  line L270 (-32, 107) -> (-17, 107) projected
  line L271 (-17, 105) -> (-30, 105) projected
  line L272 (-32, 92) -> (-32, 7.5) projected
  line L273 (-32, 7.5) -> (-32, 92) projected
  line L274 (-32, 92) -> (-32, 107) projected
  line L275 (32, 92) -> (32, 107) projected
  line L276 (30, 92) -> (32, 92) projected
  line L277 (30, 105) -> (30, 92) projected
  line L278 (17, 105) -> (30, 105) projected
  line L279 (32, 107) -> (17, 107) projected
  line L280 (17, 107) -> (17, 105) projected
  line L281 (17, 105) -> (17, 107) projected
  line L282 (-17, 107) -> (-32, 107) projected
  line L283 (-17, 105) -> (-17, 107) projected
  line L284 (-30, 105) -> (-17, 105) projected
  line L285 (-30, 92) -> (-30, 105) projected
  line L286 (-32, 107) -> (-32, 92) projected
  line L287 (32, 7.5) -> (30, 7.5) projected
  line L288 (30, 7.5) -> (32, 7.5) projected
  line L289 (32, 7.5) -> (30, 7.5) projected
  line L290 (-30, 7.5) -> (-32, 7.5) projected
  line L291 (-32, 7.5) -> (-30, 7.5) projected
  line L292 (-30, 7.5) -> (-32, 7.5) projected
  line L293 (-32, 92) -> (-30, 92) projected
  line L294 (-30, 92) -> (-32, 92) projected
  line L295 (-30, 92) -> (-32, 92) projected
  line L296 (-32, 92) -> (-30, 92) projected
  line L297 (32, 92) -> (30, 92) projected
  line L298 (30, 92) -> (32, 92) projected
  line L299 (-17, 107) -> (-32, 107) projected
  line L300 (17, 107) -> (-17, 107) projected
  line L301 (32, 107) -> (17, 107) projected
  line L302 (17, 107) -> (32, 107) projected
  line L303 (-17, 107) -> (17, 107) projected
  line L304 (-32, 107) -> (-17, 107) projected
  line L305 (-30, 105) -> (30, 105) projected
  line L306 (-17, 105) -> (-30, 105) projected
  line L307 (17, 105) -> (-17, 105) projected
  line L308 (30, 105) -> (17, 105) projected
  line L309 (-32, 7.5) -> (-30, 7.5) projected
  line L310 (-17, 107) -> (-17, 105) projected
  line L311 (-17, 107) -> (-17, 105) projected
  line L312 (-17, 107) -> (-17, 105) projected
  line L313 (-32, 7.5) -> (-30, 7.5) projected
  line L314 (30, 7.5) -> (32, 7.5) projected
  line L315 (30, 7.5) -> (32, 7.5) projected
  line L316 (30, 7.5) -> (32, 7.5) projected
  line L317 (-32, 7.5) -> (-30, 7.5) projected
  line L318 (30, 7.5) -> (32, 7.5) projected
  line L319 (-32, 7.5) -> (-30, 7.5) projected
  line L320 (-32, 7.5) -> (-30, 7.5) projected
  line L321 (-32, 7.5) -> (-30, 7.5) projected
  line L322 (-32, 7.5) -> (-32, 92) projected
  line L323 (-30, 92) -> (-32, 92) projected
  line L324 (-30, 92) -> (-30, 7.5) projected
  line L325 (32, 92) -> (30, 92) projected
  line L326 (32, 92) -> (32, 7.5) projected
  line L327 (30, 7.5) -> (32, 7.5) projected
  line L328 (30, 7.5) -> (30, 92) projected
  line L329 (-30, 105) -> (-30, 92) projected
  line L330 (-30, 92) -> (-30, 105) projected
  line L331 (-17, 105) -> (-30, 105) projected
  line L332 (-30, 105) -> (-17, 105) projected
  line L333 (-17, 107) -> (-17, 105) projected
  line L334 (-17, 105) -> (-17, 107) projected
  line L335 (-32, 107) -> (-32, 92) projected
  line L336 (-32, 92) -> (-30, 92) projected
  line L337 (-30, 92) -> (-30, 105) projected
  line L338 (-30, 105) -> (-17, 105) projected
  line L339 (-17, 105) -> (-17, 107) projected
  line L340 (-17, 107) -> (-32, 107) projected
  line L341 (-17, 107) -> (-17, 105) projected
  line L342 (-30, 92) -> (-32, 92) projected
  line L343 (-30, 105) -> (-30, 92) projected
  line L344 (-30, 92) -> (-32, 92) projected
  line L345 (-32, 92) -> (-32, 107) projected
  line L346 (-32, 107) -> (-17, 107) projected
  line L347 (-17, 107) -> (-17, 105) projected
  line L348 (-17, 105) -> (-30, 105) projected
  line L349 (-30, 92) -> (-32, 92) projected
  line L350 (-30, 92) -> (-32, 92) projected
  line L351 (-30, 92) -> (-32, 92) projected
  line L352 (17, 105) -> (17, 107) projected
  line L353 (17, 107) -> (17, 105) projected
  line L354 (-25, 100) -> (25, 100) projected
  line L355 (-25, 100) -> (25, 100) projected
  line L356 (-17, 107) -> (-17, 105) projected
  line L357 (-17, 107) -> (17, 107) projected
  line L358 (17, 105) -> (17, 107) projected
  line L359 (17, 105) -> (-17, 105) projected
  line L360 (30, 105) -> (17, 105) projected
  line L361 (17, 105) -> (30, 105) projected
  line L362 (30, 92) -> (30, 105) projected
  line L363 (30, 105) -> (30, 92) projected
  line L364 (32, 107) -> (17, 107) projected
  line L365 (17, 107) -> (17, 105) projected
  line L366 (17, 105) -> (30, 105) projected
  line L367 (30, 105) -> (30, 92) projected
  line L368 (30, 92) -> (32, 92) projected
  line L369 (32, 92) -> (32, 107) projected
  line L370 (17, 105) -> (17, 107) projected
  line L371 (32, 92) -> (30, 92) projected
  line L372 (32, 92) -> (30, 92) projected
  line L373 (32, 92) -> (30, 92) projected
  line L374 (32, 92) -> (30, 92) projected
  line L375 (32, 107) -> (32, 92) projected
  line L376 (32, 92) -> (30, 92) projected
  line L377 (30, 92) -> (30, 105) projected
  line L378 (30, 105) -> (17, 105) projected
  line L379 (17, 105) -> (17, 107) projected
  line L380 (17, 107) -> (32, 107) projected
  line L381 (17, 105) -> (17, 107) projected
  line L382 (17, 105) -> (17, 107) projected
  line L383 (17, 105) -> (17, 107) projected
  line L384 (-32, -7.5) -> (-32, 7.5) projected
  line L385 (-32, 7.5) -> (-17, 7.5) projected
  line L386 (-17, 7.5) -> (-17, -7.5) projected
  line L387 (17, -7.5) -> (17, 7.5) projected
  line L388 (32, -7.5) -> (17, -7.5) projected
  line L389 (17, 7.5) -> (32, 7.5) projected
  line L390 (32, 7.5) -> (32, -7.5) projected
  line L391 (30, 105) -> (30, -105) projected
  line L392 (30, 105) -> (30, -105) projected
  line L393 (32, -107) -> (32, 107) projected
  line L394 (-30, -105) -> (-30, 105) projected
  line L395 (-30, -105) -> (-30, 105) projected
  line L396 (-32, 107) -> (-32, -107) projected
  line L397 (-30, 105) -> (30, 105) projected
  line L398 (32, 107) -> (-32, 107) projected
  line L399 (-30, 105) -> (30, 105) projected
  line L400 (-17, 92) -> (-32, 92) projected
  line L401 (-32, 107) -> (-17, 107) projected
  line L402 (-32, 92) -> (-32, 107) projected
  line L403 (-17, 107) -> (-17, 92) projected
  line L404 (17, 92) -> (32, 92) projected
  line L405 (17, 107) -> (17, 92) projected
  line L406 (32, 107) -> (17, 107) projected
  line L407 (32, 92) -> (32, 107) projected
  line L408 (30, -105) -> (-30, -105) projected
  line L409 (-32, -107) -> (32, -107) projected
  line L410 (30, -105) -> (-30, -105) projected
  line L411 (-17, -92) -> (-32, -92) projected
  line L412 (-32, -92) -> (-32, -107) projected
  line L413 (-32, -107) -> (-17, -107) projected
  line L414 (-17, -107) -> (-17, -92) projected
  line L415 (17, -92) -> (32, -92) projected
  line L416 (17, -107) -> (17, -92) projected
  line L417 (32, -92) -> (32, -107) projected
  line L418 (32, -107) -> (17, -107) projected
  line L419 (-17, -7.5) -> (-32, -7.5) projected
  point P0 (0, 0)
  point P1 (0, 0)
  point P2 (32, 0)
  point P3 (32, 0)
  point P4 (-32, 0)
  point P5 (-32, 0)
  constraints: 99 other
extrude "Extrusion5" add sketch "Sketch7" along normal blind 2 contours L0 L1 L114 L2 | L2 L385 L127 L419 | L34 L37 L24 L50 L36 L21 | L411 L127 L30 L414 L37 L34 | L127 L385 L386 L419 | L160 L143 L270 L185 L156 L135 | L135 L156 L403 L119 L127 L400 | L411 L414 L30 L127 | L127 L119 L403 L400 | L54 L39 L67 L47 L71 L23 | L416 L30 L131 L415 L39 L54 | L183 L266 L205 L180 L157 L156 | L156 L157 L404 L131 L119 L405 | L416 L415 L131 L30 | L119 L131 L404 L405 | L388 L131 L389 L6 | L6 L10 L7 L8 | L388 L387 L389 L131
chamfer "Chamfer1" distance 4 distance2 3 2 edges at (23.5, -105, 10) (30, -98.5, 10) measured on face at (23.5, -104.5, 10) measured on face at (29.5, -98.5, 10)
chamfer "Chamfer2" distance 4 distance2 3 1 edges at (30, 0, 10) measured on face at (29.5, 0, 10)
chamfer "Chamfer3" distance 4 distance2 3 2 edges at (-30, -98.5, 10) (-23.5, -105, 10) measured on face at (-29.5, -98.5, 10) measured on face at (-23.5, -104.5, 10)
chamfer "Chamfer4" distance 4 distance2 3 1 edges at (-30, 0, 10) measured on face at (-29.5, 0, 10)
chamfer "Chamfer5" distance 4 distance2 3 2 edges at (-30, 98.5, 10) (-23.5, 105, 10) measured on face at (-23.5, 104.5, 10) measured on face at (-29.5, 98.5, 10)
chamfer "Chamfer6" distance 4 distance2 3 2 edges at (23.5, 105, 10) (30, 98.5, 10) measured on face at (29.5, 98.5, 10) measured on face at (23.5, 104.5, 10)
sketch "Sketch8" plane through (0, 0, 10) normal (0, 0, -1) x (-1, 0, 0)
  circle A0 centre (21, 0) radius 1.75
  line L0 (17, -7.5) -> (17, 7.5) projected
  circle A1 centre (21, -96) radius 1.75
  circle A2 centre (21, 96) radius 1.75
  line L1 (26, 92) -> (17, 92) projected
  line L2 (17, 92) -> (17, 101) projected
  line L3 (17, -92) -> (26, -92) projected
  line L4 (17, -101) -> (17, -92) projected
  circle A3 centre (-21, -96) radius 1.75
  line L5 (-17, -92) -> (-17, -101) projected
  line L6 (-26, -92) -> (-17, -92) projected
  circle A4 centre (-21, 0) radius 1.75
  line L7 (-17, 7.5) -> (-17, -7.5) projected
  circle A5 centre (-21, 96) radius 1.75
  line L8 (-17, 92) -> (-26, 92) projected
  line L9 (-17, 101) -> (-17, 92) projected
  point P0 (0, 0)
  point P1 (17, 0)
  dimension "d42" = 3.5
  dimension "d43" = 4
  dimension "d44" = 3.5
  dimension "d45" = 3.5
  dimension "d46" = 4
  dimension "d47" = 4
  dimension "d48" = 4
  dimension "d49" = 4
  dimension "d50" = 3.5
  dimension "d51" = 4
  dimension "d52" = 4
  dimension "d53" = 3.5
  dimension "d54" = 4
  dimension "d55" = 3.5
  dimension "d56" = 4
  dimension "d57" = 4
  constraints: 6 centre point, 2 horizontal alignment, 1 midpoint
  measures "d42" diameter of A0
  measures "d43" distance of point (17, 0) A0.centre
  measures "d44" diameter of A1
  measures "d45" diameter of A2
  measures "d46" distance from line of L1 A2.centre
  measures "d47" distance from line of L2 A2.centre
  measures "d48" distance from line of L3 A1.centre
  measures "d49" distance from line of L4 A1.centre
  measures "d50" diameter of A3
  measures "d51" distance from line of L5 A3.centre
  measures "d52" distance from line of L6 A3.centre
  measures "d53" diameter of A4
  measures "d54" distance from line of L7 A4.centre
  measures "d55" diameter of A5
  measures "d56" distance from line of L8 A5.centre
  measures "d57" distance from line of L9 A5.centre
extrude "Extrusion6" cut sketch "Sketch8" against normal up to surface (2 mm away)
body "Solid1"
